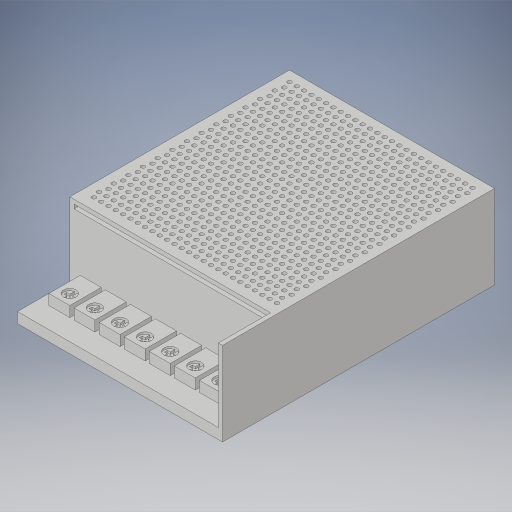
# Autodesk Inventor part: BT501_trajan20_21
Saved by Autodesk Inventor 2023 (Build 270158000, 158)
## iProperties
Company: HTBLA Kaindorf
RuleStatus: InUse
Created: 2022-10-30
Part Number: BT501_trajan20_21
Project: Zeichenmaschine_neu
Material: Generisch
Description: Netzteil
Document SubType Name: Modeling
Designer: trajan20
Density: 1 g/cm^3
Appearance: Vorgabe
Mass: 407.011 g
Surface Area: 690.643 cm^2
Volume: 407.011 cm^3
AfterDocNew0: iProperties-Editor_aufrufen
Author: jan
Keywords: 2021
Autodesk Inventor part; units mm, degrees
ref_plane "YZ Plane" through (0, 0, 0) normal (1, 0, 0) x (0, 1, 0)
ref_plane "XZ Plane" through (0, 0, 0) normal (0, 1, 0) x (-1, 0, 0)
ref_plane "XY Plane" through (0, 0, 0) normal (0, 0, 1) x (1, 0, 0)
sketch "Skizze3" plane through (0, 0, 0) normal (0, 0, 1) x (1, 0, 0)
  line L0 (0, 0) -> (-130, 0)
  line L1 (-130, 0) -> (-130, 98)
  line L2 (-130, 98) -> (0, 98)
  line L3 (0, 98) -> (0, 0)
  point P0 (-37, 30.5)
  point P1 (-78, 64.5)
  point P2 (-78, 30.5)
  dimension "d4" = 130
  dimension "d5" = 98
  dimension "d9" = 30.5
  dimension "d10" = 52
  dimension "d12" = 33.5
  dimension "d13" = 30.5
  dimension "d15" = 37
  constraints: 8 end point, 2 parallel, 1 horizontal, 1 perpendicular, 1 vertical alignment
  measures "d4" distance between parallel lines of L1 L3
  measures "d5" distance between parallel lines of L2 L0
  measures "d9" distance from line of L0 point (-78, 30.5)
  measures "d10" distance from line of L1 point (-78, 30.5)
  measures "d12" distance from line of L2 point (-78, 64.5)
  measures "d13" distance from line of L0 point (-37, 30.5)
  measures "d15" distance from line of L3 point (-37, 30.5)
extrude "Extrusion3" add sketch "Skizze3" along normal blind 40
hole "Bohrung1" at (-37, 30.5, 0) at (-78, 64.5, 0) at (-78, 30.5, 0) direction (0, 0, 1) diameter 1.7294 depth 4 tip angle 118 thread size "M2x0.25" class "6H" standard "ISO Metric profile"
sketch "Skizze4" plane through (0, 0, 40) normal (0, 0, 1) x (1, 0, 0)
  line L0 (-130, 0) -> (0, 0) projected
  line L1 (0, 0) -> (-25, 0)
  line L2 (-25, 0) -> (-25, 96)
  line L3 (-25, 96) -> (0, 96)
  line L4 (0, 96) -> (0, 0)
  line L5 (0, 98) -> (-130, 98) projected
  dimension "d23" = 25
  dimension "d26" = 2
  constraints: 8 end point, 2 parallel, 1 horizontal, 1 perpendicular
  measures "d23" distance between parallel lines of L4 L2
  measures "d26" distance between parallel lines of L3 L5
extrude "Extrusion4" cut sketch "Skizze4" against normal blind 35
sketch "Skizze5" plane through (0, 0, 5) normal (0, 0, 1) x (1, 0, 0)
  line L0 (-25, 0) -> (-25, 96) projected
  line L1 (-25, 5) -> (-10, 5)
  line L2 (-10, 5) -> (-10, 15)
  line L3 (-10, 15) -> (-25, 15)
  line L4 (-25, 15) -> (-25, 5)
  circle A0 centre (-15, 10) radius 3
  line L5 (-12.0828, 10.7) -> (-17.9172, 10.7)
  line L6 (-12.0828, 9.3) -> (-17.9172, 9.3)
  line L7 (-15.7, 9.3) -> (-15.7, 7.9)
  line L8 (-15.7, 7.9) -> (-14.3, 7.9)
  line L9 (-14.3, 7.9) -> (-14.3, 9.3)
  line L10 (-14.3, 10.7) -> (-14.3, 12.1)
  line L11 (-14.3, 12.1) -> (-15.7, 12.1)
  line L12 (-15.7, 12.1) -> (-15.7, 10.7)
  point P0 (0, 0)
  point P1 (-25, 15)
  point P2 (-10, 10)
  point P3 (-15, 9.3)
  point P4 (-15, 7.9)
  point P5 (-15, 12.1)
  point P6 (-15, 10.7)
  dimension "d29" = 15
  dimension "d30" = 10
  dimension "d31" = 15
  dimension "d34" = 5
  dimension "d35" = 6
  dimension "d36" = 1.4
  dimension "d37" = 1.4
  dimension "d38" = 1.4
  dimension "d39" = 1.4
  dimension "d40" = 1.4
  constraints: 24 end point, 5 midpoint, 5 perpendicular, 5 point on line, 4 point on circle, 3 horizontal, 3 parallel, 2 vertical, 2 vertical alignment, 1 centre point, 1 coincident, 1 horizontal alignment
  measures "d29" distance between parallel lines of L2 L0
  measures "d30" distance between parallel lines of L1 L3
  measures "d31" distance from line of point (0, 0) L3
  measures "d34" distance from line of L2 point (-15, 10)
  measures "d35" diameter of A0
  measures "d36" distance between parallel lines of L6 L5
  measures "d37" distance between parallel lines of L5 L11
  measures "d38" distance between parallel lines of L8 L6
  measures "d39" distance between parallel lines of L9 L7
  measures "d40" distance between parallel lines of L12 L10
extrude "Extrusion5" add sketch "Skizze5" along normal blind 5 contours L0 L3 L2 L1 | A0 L6 L5 | L5 L10 L11 L12 A0 | A0 L6 L7 L8 L9 | L5 L12 L11 L10 | L9 L8 L7 L6
sketch "Skizze6" plane through (0, 0, 10) normal (0, 0, 1) x (1, 0, 0)
  line L0 (-25, 0) -> (-25, 96)
  line L1 (-25, 5) -> (-10, 5)
  line L2 (-10, 5) -> (-10, 15)
  line L3 (-10, 15) -> (-25, 15)
  line L4 (-25, 15) -> (-25, 5)
  circle A0 centre (-15, 10) radius 3
  line L5 (-12.0828, 10.7) -> (-17.9172, 10.7)
  line L6 (-12.0828, 9.3) -> (-17.9172, 9.3)
  line L7 (-15.7, 9.3) -> (-15.7, 7.9)
  line L8 (-15.7, 7.9) -> (-14.3, 7.9)
  line L9 (-14.3, 7.9) -> (-14.3, 9.3)
  line L10 (-14.3, 10.7) -> (-14.3, 12.1)
  line L11 (-14.3, 12.1) -> (-15.7, 12.1)
  line L12 (-15.7, 12.1) -> (-15.7, 10.7)
  line L13 (0, 0) -> (-25, 0) projected
  point P0 (0, -5)
  point P1 (-10, 10)
  point P2 (-15, 9.3)
  point P3 (-15, 7.9)
  point P4 (-15, 12.1)
  point P5 (-15, 10.7)
  dimension "d41" = 15
  dimension "d42" = 10
  dimension "d43" = 20
  dimension "d44" = 5
  dimension "d45" = 6
  dimension "d46" = 1.4
  dimension "d47" = 1.4
  dimension "d48" = 1.4
  dimension "d49" = 1.4
  dimension "d50" = 1.4
  dimension "d51" = 5
  constraints: 26 end point, 5 midpoint, 5 perpendicular, 5 point on line, 4 point on circle, 3 horizontal, 3 parallel, 2 vertical, 2 vertical alignment, 1 centre point, 1 coincident, 1 horizontal alignment, 1 other
  measures "d41" distance between parallel lines of L2 L0
  measures "d42" distance between parallel lines of L1 L3
  measures "d43" distance from line of point (0, -5) L3
  measures "d44" distance from line of L2 point (-15, 10)
  measures "d45" diameter of A0
  measures "d46" distance between parallel lines of L6 L5
  measures "d47" distance between parallel lines of L5 L11
  measures "d48" distance between parallel lines of L8 L6
  measures "d49" distance between parallel lines of L9 L7
  measures "d50" distance between parallel lines of L12 L10
  measures "d51" distance of the line from the sketch origin of L1
extrude "Extrusion6" cut sketch "Skizze6" against normal blind 1 contours A0 L6 L5 | L5 L10 L11 L12 A0 | A0 L6 L7 L8 L9 | L5 L12 L11 L10 | L9 L8 L7 L6
extrude "Extrusion7" cut sketch "Skizze6" against normal blind 2 contours A0 L6 L5 | L5 L12 L11 L10 | L9 L8 L7 L6
pattern_linear "Rechteckige Anordnung1" count 7 spacing 12 along (0, 1, 0) of "Extrusion5", "Extrusion7", "Extrusion6"
sketch "Skizze7" plane through (-25, 0, 40) normal (1, 0, 0) x (0, 0, -1)
  line L0 (2, 2) -> (4, 2)
  line L1 (4, 2) -> (4, 94)
  line L2 (4, 94) -> (2, 94)
  line L3 (2, 94) -> (2, 2)
  line L4 (0, 0) -> (0, 96) projected
  line L5 (35, 0) -> (0, 0) projected
  line L6 (0, 96) -> (35, 96) projected
  point P0 (40, 0)
  dimension "d59" = 2
  dimension "d60" = 2
  dimension "d61" = 2
  dimension "d62" = 2
  constraints: 8 end point, 2 parallel, 1 horizontal, 1 perpendicular
  measures "d59" distance between parallel lines of L4 L3
  measures "d60" distance between parallel lines of L5 L0
  measures "d61" distance between parallel lines of L3 L1
  measures "d62" distance between parallel lines of L6 L2
extrude "Extrusion8" cut sketch "Skizze7" against normal blind 103
sketch "Skizze8" plane through (0, 0, 40) normal (0, 0, 1) x (1, 0, 0)
  circle A0 centre (-125, 5) radius 1
  line L0 (-130, 98) -> (-130, 0) projected
  line L1 (-130, 0) -> (-25, 0) projected
  circle A1 centre (-121.5, 6) radius 1
  circle A2 centre (-125, 8.5) radius 1
  circle A3 centre (-121.5, 9.5) radius 1
  point P0 (0, 0)
  dimension "d65" = 2
  dimension "d66" = 5
  dimension "d67" = 5
  dimension "d68" = 2
  dimension "d69" = 3.5
  dimension "d70" = 1
  dimension "d71" = 2
  dimension "d72" = 3.5
  dimension "d73" = 2
  dimension "d74" = 3.5
  constraints: 4 centre point, 2 vertical alignment
  measures "d65" diameter of A0
  measures "d66" distance from line of L0 A0.centre
  measures "d67" distance from line of L1 A0.centre
  measures "d68" diameter of A1
  measures "d69" horizontal distance of A0.centre A1.centre
  measures "d70" vertical distance of A1.centre A0.centre
  measures "d71" diameter of A2
  measures "d72" distance of A0.centre A2.centre
  measures "d73" diameter of A3
  measures "d74" distance of A1.centre A3.centre
extrude "Extrusion9" cut sketch "Skizze8" against normal blind 2
pattern_linear "Rechteckige Anordnung2" count 13 spacing 7 along (0, 1, 0) count 14 spacing 7 along (1, 0, 0) of "Extrusion9"
equation "\"d9\" = d13"
equation "\"d38\" = d37"
equation "\"d40\" = d39"
equation "\"d48\" = d47"
equation "\"d50\" = d49"
equation "\"d68\" = d65"
equation "\"d70\" = 0.5 * d65"
